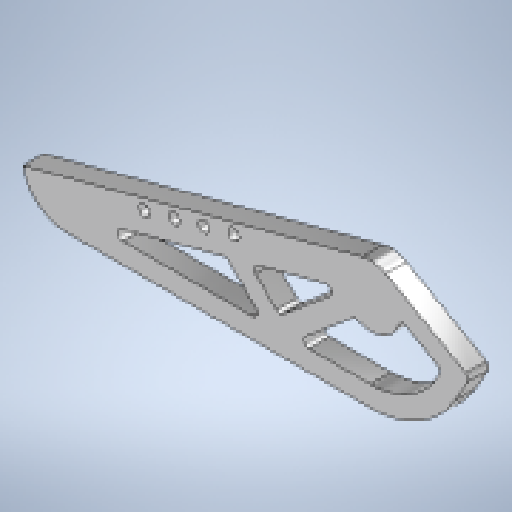
# Autodesk Inventor part: Arms
Saved by Autodesk Inventor 2023.2 (Build 272271000, 271)
## iProperties
Created: 2024-01-12
Part Number: Arms
Material: Aluminum 6061
Document SubType Name: Modeling
Designer: Nathan Cai
Mass: 38.5716 g
Surface Area: 83.6669 cm^2
Volume: 14.2858 cm^3
Density: 2.7 g/cm^3
Appearance: Aluminum - Flat
Author: Nathan Cai
Autodesk Inventor part; units mm, degrees
ref_plane "YZ Plane" through (0, 0, 0) normal (1, 0, 0) x (0, 1, 0)
ref_plane "XZ Plane" through (0, 0, 0) normal (0, 1, 0) x (-1, 0, 0)
ref_plane "XY Plane" through (0, 0, 0) normal (0, 0, 1) x (1, 0, 0)
sketch "Sketch1" plane through (0, 0, 0) normal (0, 0, 1) x (1, 0, 0)
  circle A0 centre (0, 0) radius 3.175
  arc A1 (0, -30.1625) -> (26.1215, -15.0812) centre (0, 0) ccw
  arc A2 (7.1237, 6.3228) -> (-2.4653, 9.2004) centre (0, 0) ccw
  line L0 (0, -30.1625) -> (-94.3629, -30.1625)
  circle A3 centre (0, 0) radius 109.3391 construction
  line L1 (0, 0) -> (0, -30.1625) construction
  line L2 (-2.4653, 9.2004) -> (-107.6772, -18.991)
  arc A4 (-107.6772, -18.991) -> (-94.3629, -30.1625) centre (-94.3629, -16.6428) ccw
  line L3 (-88.8695, -23.8125) -> (3.0668, 0.8218)
  line L4 (1.5875, 2.7496) -> (22.0256, -9.0503)
  arc A5 (0, -23.8125) -> (22.0256, -9.0503) centre (0, 0) ccw
  line L5 (0, -23.8125) -> (-88.8695, -23.8125)
  circle A6 centre (0, 0) radius 9.525
  line L6 (-44.7031, -11.9782) -> (-32.8688, -23.8125)
  line L7 (-37.6206, -10.0804) -> (-28.1908, -19.5102)
  line L8 (-28.1908, -19.5102) -> (-8.9201, -3.3402)
  line L9 (-23.4392, -23.8125) -> (-4.8384, -8.2046)
  line L10 (0, 0) -> (26.1215, -15.0812) construction
  line L11 (26.1215, -15.0812) -> (30.884, -6.8324)
  line L12 (30.884, -6.8324) -> (4.7625, 8.2489)
  circle A7 centre (-42.4523, -4.8011) radius 1.7526
  line L13 (-7.2966, -6.1226) -> (-28.3786, -23.8125) construction
  line L14 (-8.5011, 4.2961) -> (-106.7618, -22.0327) construction
  line L15 (-28.3786, -23.8125) -> (-41.1618, -11.0293) construction
  line L16 (-44.6974, -8.6896) -> (-46.3409, -2.556) construction
  line L17 (-46.3409, -2.556) -> (-40.2072, -0.9125) construction
  line L18 (-40.2072, -0.9125) -> (-38.5637, -7.0461) construction
  line L19 (-38.5637, -7.0461) -> (-44.6974, -8.6896) construction
  line L20 (-44.6974, -8.6896) -> (-40.2072, -0.9125) construction
  line L21 (-46.3409, -2.556) -> (-38.5637, -7.0461) construction
  line L22 (-109.2456, -13.1377) -> (-104.1652, -32.098) construction
  circle A8 centre (-51.6528, -7.2663) radius 1.7526
  circle A9 centre (-60.8532, -9.7316) radius 1.7526
  circle A10 centre (-70.0536, -12.1968) radius 1.7526
  point P0 (-105.7272, -23.9664)
  point P1 (9.3646, -1.7405)
  point P2 (-9.2004, -2.4653)
  point P3 (-12.9484, -3.4695)
  dimension "d22" = 218.6781
  dimension "d0" = 6.35
  dimension "d2" = 19.05
  dimension "d12" = 15
  dimension "d13" = 30.1625
  dimension "d14" = 9.525
  dimension "d21" = 6.35
  dimension "d23" = 60
  dimension "d25" = 9.525
  dimension "d29" = 3.5052
  dimension "d30" = 6.35
  dimension "d31" = 6.35
  dimension "d33" = 45
  dimension "d35" = 3.175
  dimension "d36" = 25
  dimension "d37" = 3.175
  dimension "d42" = 3.175
  dimension "d50" = 6.35
  dimension "d51" = 69.85
  dimension "d54" = 9.525
  constraints: 46 end point, 17 point on circle, 10 centre point, 10 point on line, 8 parallel, 7 tangent, 6 coincident, 3 perpendicular, 2 midpoint, 1 concentric, 1 horizontal, 11 other
  measures "d0" diameter of A0
  measures "d2" diameter of A2
  measures "d12" angle of L0 L2
  measures "d13" radius of A1
  measures "d14" distance between parallel lines of L2 L3
  measures "d21" distance between parallel lines of L0 L5
  measures "d23" angle of L1 L10
  measures "d25" distance from line of L11.end L10
  measures "d29" diameter of A7
  measures "d30" distance between parallel lines of L9 L8
  measures "d31" distance between parallel lines of L6 L7
  measures "d33" angle of L5 L6
  measures "d35" distance between parallel lines of L8 L13
  measures "d36" angle of L3 L8
  measures "d37" distance between parallel lines of L2 L14
  measures "d42" distance between parallel lines of L15 L7
  measures "d50" distance of L16.end L17.end
  measures "d51" distance between parallel lines of L18 L22
  measures "d54" distance of A7.centre A8.centre
extrude "Extrusion1" add sketch "Sketch1" along normal blind 6.35 contours A0 L3 | A0 L4 A6 L3 | L3 A0 | L3 A6 A2 L4 A0 | L3 L5 A5 L4 A6 A2 L12 L11 A1 L0 A4 L2 | L7 L8 A6 L9 L5 L6 L3
fillet "Fillet2" radius 1.5875 12 edges at (-44.7031, -11.9782, 3.175) (-32.8688, -23.8125, 3.175) (-28.1908, -19.5102, 3.175) (-37.6206, -10.0804, 3.175) (-9.2004, -2.4653, 3.175) (-8.9201, -3.3402, 3.175) (-4.8384, -8.2046, 3.175) (-23.4392, -23.8125, 3.175) (9.3646, -1.7405, 3.175) (22.0256, -9.0503, 3.175) (-88.8695, -23.8125, 3.175) (30.884, -6.8324, 3.175)
equation "\"d22\" = 7.25 * d13"
body "Solid1"
